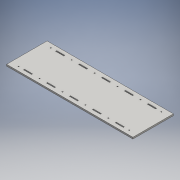
# Autodesk Inventor part: BASE
Saved by Autodesk Inventor 2016 (Build 200138000, 138)
## iProperties
Created: 2017-09-06
Part Number: BASE
Material: Genérico
Document SubType Name: Modeling
Designer: Alumno
Density: 1 g/cm^3
Appearance: Valor por defecto
Author: Alumno
Autodesk Inventor part; units mm, degrees
ref_plane "YZ Plane" through (0, 0, 0) normal (1, 0, 0) x (0, 1, 0)
ref_plane "XZ Plane" through (0, 0, 0) normal (0, 1, 0) x (-1, 0, 0)
ref_plane "XY Plane" through (0, 0, 0) normal (0, 0, 1) x (1, 0, 0)
sketch "Boceto1" plane through (0, 0, 0) normal (0, 0, 1) x (1, 0, 0)
  line L0 (0, 4) -> (0, 0)
  line L1 (0, -114.3085) -> (0, -115)
  circle A0 centre (27.5, 2) radius 1.8
  circle A1 centre (27.5, -117) radius 1.8
  circle A2 centre (112.5, -117) radius 1.8
  circle A3 centre (197.5, 2) radius 1.8
  circle A4 centre (112.5, 2) radius 1.8
  circle A5 centre (197.5, -117) radius 1.8
  circle A6 centre (282.5, 2) radius 1.8
  circle A7 centre (282.5, -117) radius 1.8
  circle A8 centre (360, 2) radius 1.8
  circle A9 centre (360, -117) radius 1.8
  line L2 (-74, 12.5) -> (384, 12.5)
  line L3 (384, 12.5) -> (384, -127.5)
  line L4 (384, -127.5) -> (-74, -127.5)
  line L5 (-74, -127.5) -> (-74, 12.5)
  line L6 (389, 17.5) -> (-79, 17.5)
  line L7 (-79, 17.5) -> (-79, -132.5)
  line L8 (-79, -132.5) -> (389, -132.5)
  line L9 (389, -132.5) -> (389, 17.5)
  circle A10 centre (-50, -117) radius 1.8
  circle A11 centre (-50, 2) radius 1.8
  point P0 (-74, -127.5)
  point P1 (385, 4)
  dimension "d0" = 3.6
  dimension "d1" = 3.6
  dimension "d2" = 3.6
  dimension "d3" = 3.6
  dimension "d4" = 3.6
  dimension "d5" = 3.6
  dimension "d7" = 3.6
  dimension "d8" = 3.6
  dimension "d9" = 3.6
  dimension "d11" = 3.6
  dimension "d12" = 3.6
  constraints: 20 end point, 12 centre point, 4 parallel, 2 perpendicular, 1 horizontal, 3 other
  measures "d0" diameter of A0
  measures "d1" diameter of A1
  measures "d2" diameter of A2
  measures "d3" diameter of A3
  measures "d4" diameter of A4
  measures "d5" diameter of A5
  measures "d7" diameter of A7
  measures "d8" diameter of A8
  measures "d9" diameter of A9
  measures "d11" diameter of A10
  measures "d12" diameter of A11
extrude "Extrusión1" add sketch "Boceto1" along normal blind 6 contours L2 L3 L4 L5 | L9 L8 L7 L6
sketch "Boceto2" plane through (0, 0, 6) normal (0, 0, 1) x (1, 0, 0)
  line L0 (55, 0) -> (55, 4)
  line L1 (0, 4) -> (0, 0)
  line L2 (-30, 4) -> (-30, 0)
  line L3 (-70, 12.5) -> (-70, -127.5)
  line L4 (-30, -119) -> (-30, -115)
  line L5 (55, -119) -> (55, -115)
  line L6 (0, -119) -> (0, -115)
  line L7 (85, -119) -> (85, -115)
  line L8 (140, -119) -> (140, -115)
  line L9 (170, -119) -> (170, -115)
  line L10 (225, -119) -> (225, -115)
  line L11 (170, 4) -> (170, 0)
  line L12 (225, 4) -> (225, 0)
  line L13 (255, 4) -> (255, 0)
  line L14 (310, 4) -> (310, 0)
  line L15 (255, -119) -> (255, -115)
  line L16 (310, -119) -> (310, -115)
  line L17 (340, 4) -> (340, 0)
  line L18 (380, 0) -> (380, 4)
  line L19 (340, -119) -> (340, -115)
  line L20 (380, -127.5) -> (380, 12.5)
  circle A0 centre (27.5, 2) radius 1.8
  circle A1 centre (27.5, -117) radius 1.8
  circle A2 centre (112.5, -117) radius 1.8
  circle A3 centre (197.5, 2) radius 1.8
  line L21 (85, 4) -> (85, 0)
  line L22 (140, 4) -> (140, 0)
  circle A4 centre (112.5, 2) radius 1.8
  circle A5 centre (197.5, -117) radius 1.8
  circle A6 centre (282.5, 2) radius 1.8
  circle A7 centre (282.5, -117) radius 1.8
  circle A8 centre (360, 2) radius 1.8
  circle A9 centre (360, -117) radius 1.8
  line L23 (384, 12.5) -> (384, -127.5)
  line L24 (384, -127.5) -> (-74, -127.5)
  line L25 (-74, -127.5) -> (-74, 12.5)
  line L26 (389, 17.5) -> (-79, 17.5)
  line L27 (-79, 17.5) -> (-79, -132.5)
  line L28 (-79, -132.5) -> (389, -132.5)
  line L29 (389, -132.5) -> (389, 17.5)
  circle A10 centre (-50, -117) radius 1.8
  circle A11 centre (-50, 2) radius 1.8
  line L30 (-30, 4) -> (0, 4)
  line L31 (0, 4) -> (0, 0)
  line L32 (0, 0) -> (-30, 0)
  line L33 (-30, 0) -> (-30, 4)
  line L34 (55, 4) -> (85, 4)
  line L35 (85, 4) -> (85, 0)
  line L36 (85, 0) -> (55, 0)
  line L37 (55, 0) -> (55, 4)
  line L38 (140, 4) -> (170, 4)
  line L39 (170, 4) -> (170, 0)
  line L40 (170, 0) -> (140, 0)
  line L41 (140, 0) -> (140, 4)
  line L42 (225, 4) -> (255, 4)
  line L43 (255, 4) -> (255, 0)
  line L44 (255, 0) -> (225, 0)
  line L45 (225, 0) -> (225, 4)
  line L46 (310, 4) -> (340, 4)
  line L47 (340, 4) -> (340, 0)
  line L48 (340, 0) -> (310, 0)
  line L49 (310, 0) -> (310, 4)
  line L50 (-30, -119) -> (0, -119)
  line L51 (0, -119) -> (0, -115)
  line L52 (0, -115) -> (-30, -115)
  line L53 (-30, -115) -> (-30, -119)
  line L54 (55, -115) -> (85, -115)
  line L55 (85, -115) -> (85, -119)
  line L56 (85, -119) -> (55, -119)
  line L57 (55, -119) -> (55, -115)
  line L58 (140, -115) -> (170, -115)
  line L59 (170, -115) -> (170, -119)
  line L60 (170, -119) -> (140, -119)
  line L61 (140, -119) -> (140, -115)
  line L62 (225, -115) -> (255, -115)
  line L63 (255, -115) -> (255, -119)
  line L64 (255, -119) -> (225, -119)
  line L65 (225, -119) -> (225, -115)
  line L66 (310, -115) -> (340, -115)
  line L67 (340, -115) -> (340, -119)
  line L68 (340, -119) -> (310, -119)
  line L69 (310, -119) -> (310, -115)
  point P0 (-74, -127.5)
  point P1 (385, 4)
  dimension "d15" = 3.6
  dimension "d16" = 3.6
  dimension "d17" = 3.6
  dimension "d18" = 3.6
  dimension "d19" = 3.6
  dimension "d20" = 3.6
  dimension "d22" = 3.6
  dimension "d23" = 3.6
  dimension "d24" = 3.6
  dimension "d26" = 3.6
  dimension "d27" = 3.6
  constraints: 140 end point, 23 parallel, 12 centre point, 11 perpendicular, 10 horizontal, 2 other
  measures "d15" diameter of A0
  measures "d16" diameter of A1
  measures "d17" diameter of A2
  measures "d18" diameter of A3
  measures "d19" diameter of A4
  measures "d20" diameter of A5
  measures "d22" diameter of A7
  measures "d23" diameter of A8
  measures "d24" diameter of A9
  measures "d26" diameter of A10
  measures "d27" diameter of A11
extrude "Extrusión2" cut sketch "Boceto2" against normal blind 6 contours L0 L34 L21 L36 | L1 L32 L2 L30 | L4 L52 L6 L50 | L5 L54 L7 L56 | L8 L58 L9 L60 | L10 L62 L15 L64 | L11 L40 L22 L38 | L42 L13 L44 L12 | L46 L17 L48 L14 | L16 L66 L19 L68
